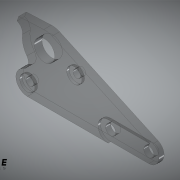
# Autodesk Inventor part: ロッド根本２
Saved by Autodesk Inventor 2020 (Build 240168000, 168)
## iProperties
Created: 2019-12-03
Part Number: ロッド根本２
Material: ポリカーボネート、クリア
Document SubType Name: Modeling
Designer: tanjihayato
Density: 1.2 g/cm^3
Appearance: ポリカーボネート - クリア
Mass: 2.90279 g
Surface Area: 23.7672 cm^2
Volume: 2.41899 cm^3
Author: tanjihayato
Autodesk Inventor part; units mm, degrees
ref_plane "YZ Plane" through (0, 0, 0) normal (1, 0, 0) x (0, 1, 0)
ref_plane "XZ Plane" through (0, 0, 0) normal (0, 1, 0) x (-1, 0, 0)
ref_plane "XY Plane" through (0, 0, 0) normal (0, 0, 1) x (1, 0, 0)
sketch "スケッチ2" plane through (0, 0, 0) normal (0, 0, 1) x (1, 0, 0)
  circle A0 centre (0, 0) radius 2
  circle A1 centre (15, 0) radius 2
  arc A2 (-0.2273, 4.9948) -> (-2.9263, -4.0542) centre (0, 0) ccw
  circle A3 centre (55, 0) radius 1.5
  circle A4 centre (55, 0) radius 4.025
  arc A5 (57.9262, 6.3865) -> (54.6807, 7.0177) centre (55, 0) ccw
  arc A6 (46.6204, -10.301) -> (48.0377, -5.2999) centre (45.4517, -7.2684) ccw
  circle A7 centre (95, -15) radius 2
  circle A8 centre (80, -15) radius 2
  arc A9 (95, -19) -> (96.6662, -11.3635) centre (95, -15) ccw
  line L0 (48.2385, -19) -> (80, -19)
  line L1 (57.9262, 6.3865) -> (96.6662, -11.3635)
  arc A10 (46.3293, 1.1755) -> (48.0377, -5.2999) centre (55, 0) ccw
  arc A11 (62.367, -1.4063) -> (54.6591, 7.4922) centre (55, 0) ccw
  line L2 (-0.2273, 4.9948) -> (54.6591, 7.4922)
  circle A12 centre (13, -10) radius 1.5
  arc A13 (10.3663, -13.6488) -> (12.3637, -14.4548) centre (13, -10) ccw
  line L3 (-2.9263, -4.0542) -> (10.3663, -13.6488)
  arc A14 (54.3637, -20.4538) -> (59.4202, -16.8428) centre (55, -15.999) ccw
  line L4 (12.3637, -14.4548) -> (54.3637, -20.4538)
  line L5 (59.4202, -16.8428) -> (62.367, -1.4063)
  circle A15 centre (66.7169, -2.5911) radius 1.5
  circle A16 centre (66.7169, -2.5911) radius 4.5 construction
  circle A17 centre (48.2385, -14.5) radius 1.5
  arc A18 (46.6204, -10.301) -> (48.2385, -19) centre (48.2385, -14.5) ccw
  line L6 (358.0202, -11) -> (380, -19)
  circle A19 centre (348.0202, -15) radius 1.25
  circle A20 centre (333.0202, -15) radius 1.25
  circle A21 centre (318.0202, -15) radius 1.25
  circle A22 centre (303.0202, -15) radius 1.25
  line L7 (80, -11) -> (207.8755, -11)
  line L8 (358.0202, -11) -> (248.9511, -11)
  arc A23 (213.7823, -10) -> (213.8378, -11) centre (210.8567, -10.6639) ccw
  line L9 (213.7823, -10) -> (214.7761, -9.8894)
  line L10 (213.8378, -11) -> (214.8378, -11)
  line L11 (219.357, -11) -> (218.357, -11)
  line L12 (218.2737, -9.5) -> (219.2676, -9.3894)
  line L13 (222.8762, -11) -> (223.8762, -11)
  line L14 (222.7652, -9) -> (223.7591, -8.8894)
  arc A24 (214.8378, -11) -> (218.357, -11) centre (216.5974, -10.3453) ccw
  arc A25 (218.2737, -9.5) -> (214.7761, -9.8894) centre (216.5974, -10.3453) ccw
  arc A26 (219.357, -11) -> (222.8762, -11) centre (221.1166, -10.0946) ccw
  arc A27 (222.7652, -9) -> (219.2676, -9.3894) centre (221.1166, -10.0946) ccw
  line L15 (210.8567, -10.6639) -> (233.0155, -9.4343) construction
  arc A28 (223.8762, -11) -> (229.892, -10.6107) centre (226.7628, -8.9308) ccw
  arc A29 (226.8407, -8.7739) -> (223.7591, -8.8894) centre (225.3075, -9.0352) ccw
  arc A30 (226.8407, -8.7739) -> (230.4998, -7.0068) centre (226.5478, -3.4953) ccw
  arc A31 (233.6316, -8.397) -> (230.4998, -7.0068) centre (231.2455, -9.5496) ccw
  arc A32 (235.4619, -12.6053) -> (229.892, -10.6107) centre (230.3136, -18.2076) ccw
  arc A33 (235.4619, -12.6053) -> (239.6511, -11) centre (234.0497, -2.6513) ccw
  arc A34 (259.6965, 4.4867) -> (265.8152, 14.9495) centre (248.2498, 18.2013) ccw
  arc A35 (220.191, -4.195) -> (265.8152, 14.9495) centre (219.3797, 61.6752) ccw
  line L16 (220.191, -4.195) -> (207.615, -4.3499)
  arc A36 (196.7777, -11) -> (207.615, -4.3499) centre (196.7777, 1.1554) ccw
  line L17 (222.8762, -11) -> (240.076, -10.0456) construction
  line L18 (222.7652, -9) -> (239.478, -8.0726) construction
  line L19 (239.6511, -11) -> (240.6511, -11)
  arc A37 (240.6511, -11) -> (242.7511, -11) centre (241.7011, -11) ccw
  line L20 (242.7511, -11) -> (243.7511, -11)
  arc A38 (243.7511, -11) -> (245.8511, -11) centre (244.8011, -11) ccw
  line L21 (245.8511, -11) -> (246.8511, -11)
  arc A39 (246.8511, -11) -> (248.9511, -11) centre (247.9011, -11) ccw
  arc A40 (240.735, -6.337) -> (238.7449, -7.0075) centre (239.7428, -6.6807) ccw
  arc A41 (243.5362, -5.2633) -> (241.5809, -6.0291) centre (242.5618, -5.6544) ccw
  arc A42 (246.2823, -4.0554) -> (244.3663, -4.9148) centre (245.3279, -4.4932) ccw
  arc A43 (248.9668, -2.7162) -> (247.0946, -3.6672) centre (248.0347, -3.1996) ccw
  arc A44 (233.6316, -8.397) -> (238.7449, -7.0075) centre (219.9279, 52.1342) ccw
  arc A45 (240.735, -6.337) -> (241.5809, -6.0291) centre (219.9279, 52.1342) ccw
  arc A46 (243.5362, -5.2633) -> (244.3663, -4.9148) centre (219.9279, 52.1342) ccw
  arc A47 (246.2823, -4.0554) -> (247.0946, -3.6672) centre (219.9279, 52.1342) ccw
  arc A48 (248.9668, -2.7162) -> (259.6965, 4.4867) centre (219.9279, 52.1342) ccw
  line L22 (196.7777, -11) -> (196.7777, -15)
  circle A49 centre (200.7777, -15) radius 1.25
  circle A50 centre (215.7777, -15) radius 1.25
  arc A51 (196.7777, -15) -> (200.7777, -19) centre (200.7777, -15) ccw
  arc A52 (215.7777, -19) -> (217.9536, -11.6436) centre (215.7777, -15) ccw
  circle A53 centre (200.7777, -15) radius 1.5
  circle A54 centre (215.7777, -15) radius 1.5
  line L23 (200.7777, -19) -> (215.7777, -19)
  circle A55 centre (45.4517, -7.2684) radius 1.5
  arc A56 (46.3293, 1.1755) -> (44.1782, 4.6812) centre (43.1088, 1.6121) ccw
  line L24 (54.6807, 7.0177) -> (44.8362, 6.5698)
  line L25 (44.8362, 6.5698) -> (44.1782, 4.6812)
  line L26 (80, -19) -> (95, -19)
  dimension "d81" = 4
  dimension "d82" = 4
  dimension "d83" = 15
  dimension "d84" = 3
  dimension "d85" = 3
  dimension "d86" = 8.05
  dimension "d87" = 3
  dimension "d88" = 6.5
  dimension "d89" = 4
  dimension "d90" = 4
  dimension "d91" = 15
  dimension "d92" = 15
  dimension "d93" = 3
  dimension "d94" = 3
  dimension "d95" = 3
  dimension "d96" = 40
  dimension "d97" = 40
  dimension "d98" = 15
  dimension "d99" = 13
  dimension "d100" = 3
  dimension "d101" = 3
  dimension "d102" = 3
  dimension "d104" = 380
  dimension "d106" = 4
  dimension "d108" = 2.5
  dimension "d109" = 2.5
  dimension "d110" = 2.5
  dimension "d111" = 2.5
  dimension "d113" = 15
  dimension "d114" = 15
  dimension "d115" = 15
  dimension "d116" = 10
  dimension "d117" = 6
  dimension "d118" = 1
  dimension "d119" = 1.5
  dimension "d120" = 1
  dimension "d121" = 1
  dimension "d122" = 1
  dimension "d123" = 2
  dimension "d124" = 1
  dimension "d125" = 1.0015
  dimension "d126" = 1.0015
  dimension "d127" = 0.7511
  dimension "d128" = 0.7511
  dimension "d129" = 3.176
  dimension "d130" = 3.176
  dimension "d131" = 1.05
  dimension "d132" = 1.05
  dimension "d133" = 1.05
  dimension "d134" = 1
  dimension "d135" = 1
  dimension "d136" = 1
  dimension "d137" = 2.1
  dimension "d138" = 2.1
  dimension "d139" = 2.1
  dimension "d140" = 2.1
  dimension "d141" = 3
  dimension "d142" = 3
  dimension "d143" = 3
  dimension "d144" = 2.5
  dimension "d145" = 2.5
  dimension "d146" = 15
  dimension "d148" = 8
  dimension "d149" = 8
  constraints: 87 point on circle, 57 centre point, 54 end point, 25 tangent, 13 point on line, 10 coincident, 8 horizontal, 7 collinear, 6 horizontal alignment, 2 concentric, 2 parallel, 1 vertical, 1 vertical alignment, 2 other
  measures "d81" diameter of A0
  measures "d82" diameter of A1
  measures "d83" distance of point (0, 0) A1.centre
  measures "d84" radial gap between concentric circles of A0 A2
  measures "d85" diameter of A3
  measures "d86" diameter of A4
  measures "d87" radial gap between concentric circles of A4 A5
  measures "d88" diameter of A6
  measures "d89" diameter of A7
  measures "d90" diameter of A8
  measures "d91" distance of A8.centre A7.centre
  measures "d92" diameter of A11
  measures "d93" diameter of A12
  measures "d94" radial gap between concentric circles of A12 A13
  measures "d95" diameter of A15
  measures "d96" distance of A4.centre A1.centre
  measures "d97" horizontal distance of A3.centre A7.centre
  measures "d98" vertical distance of A8.centre A3.centre
  measures "d99" horizontal distance of A12.centre point (0, 0)
  measures "d100" diameter of A17
  measures "d101" radial gap between concentric circles of A16 A15
  measures "d102" radial gap between concentric circles of A17 A18
  measures "d104" horizontal distance of point (0, 0) L6.end
  measures "d106" radius of A9
  measures "d108" diameter of A19
  measures "d109" diameter of A20
  measures "d110" diameter of A21
  measures "d111" diameter of A22
  measures "d113" distance of A21.centre A22.centre
  measures "d114" distance of A21.centre A20.centre
  measures "d115" distance of A19.centre A20.centre
  measures "d116" horizontal distance of A19.centre L6.start
  measures "d117" diameter of A23
  measures "d118" vertical distance of L10.start L9.start
  measures "d119" vertical distance of L11.end L12.start
  measures "d120" distance of L10.start L10.end
  measures "d121" distance of L11.end L11.start
  measures "d122" distance of L13.start L13.end
  measures "d123" vertical distance of L13.start L14.start
  measures "d124" distance of L14.start L14.end
  measures "d125" distance from line of L15 L14.start
  measures "d126" distance from line of L13.start L15
  measures "d127" distance from line of L15 L12.start
  measures "d128" distance from line of L15 L11.end
  measures "d129" angle of L14 L18
  measures "d130" angle of L13 L17
  measures "d131" radius of A37
  measures "d132" radius of A38
  measures "d133" radius of A39
  measures "d134" distance of L21.start L21.end
  measures "d135" distance of L20.start L20.end
  measures "d136" distance of L19.start L19.end
  measures "d137" diameter of A40
  measures "d138" diameter of A41
  measures "d139" diameter of A42
  measures "d140" diameter of A43
  measures "d141" distance of A40.centre A41.centre
  measures "d142" distance of A42.centre A41.centre
  measures "d143" distance of A43.centre A42.centre
  measures "d144" diameter of A49
  measures "d145" diameter of A50
  measures "d146" distance of A50.centre A49.centre
  measures "d148" diameter of A51
  measures "d149" diameter of A52
extrude "押し出し2" add sketch "スケッチ2" along normal blind 3 contours A11 L5 A14 L0 A18 A6 A10 A56 L25 L24 A5 L1 | L1 A9 L26 L0 A14 L5 A11
sketch "スケッチ3" plane through (0, 0, 3) normal (0, 0, 1) x (1, 0, 0)
  circle A0 centre (55, 0) radius 4.025 projected
  circle A1 centre (80, -15) radius 2 projected
  circle A2 centre (95, -15) radius 2 projected
  circle A3 centre (48.2385, -14.5) radius 1.5 projected
  circle A4 centre (66.7169, -2.5911) radius 1.5 projected
  arc A5 (57.9262, 6.3865) -> (54.6807, 7.0177) centre (55, 0) ccw projected
  line L0 (54.6807, 7.0177) -> (44.8362, 6.5698) projected
  line L1 (44.8362, 6.5698) -> (44.1782, 4.6812) projected
  arc A6 (46.3293, 1.1755) -> (44.1782, 4.6812) centre (43.1088, 1.6121) ccw projected
  arc A7 (46.3293, 1.1755) -> (48.0377, -5.2999) centre (55, 0) ccw projected
  arc A8 (46.6204, -10.301) -> (48.0377, -5.2999) centre (45.4517, -7.2684) ccw projected
  arc A9 (46.6204, -10.301) -> (48.2385, -19) centre (48.2385, -14.5) ccw projected
  line L2 (48.2385, -19) -> (95, -19) projected
  arc A10 (95, -19) -> (96.6662, -11.3635) centre (95, -15) ccw projected
  line L3 (96.6662, -11.3635) -> (57.9262, 6.3865) projected
  arc A11 (80, -11) -> (80, -19) centre (80, -15) ccw
  line L4 (80, -19) -> (95, -19)
  line L5 (48.2385, -19) -> (95, -19) projected
  line L6 (80, -11) -> (95.8727, -11)
  circle A12 centre (66.7169, -2.5911) radius 3
  circle A13 centre (48.2385, -14.5) radius 3
  point P0 (0, 0)
  dimension "d164" = 6
  dimension "d165" = 6
  constraints: 4 end point, 3 centre point, 3 coincident, 3 point on circle, 3 tangent, 2 horizontal, 2 point on line
  measures "d164" diameter of A12
  measures "d165" diameter of A13
extrude "押し出し3" cut sketch "スケッチ3" against normal blind 1 contours L3 A10 L2 A11 L6 | A12 | A13
sketch "スケッチ4" plane through (0, 0, 3) normal (0, 0, 1) x (1, 0, 0)
  circle A0 centre (95, -15) radius 2 projected
  circle A1 centre (80, -15) radius 2 projected
  arc A2 (95, -19) -> (96.6662, -11.3635) centre (95, -15) ccw projected
  line L0 (95.8727, -11) -> (96.6662, -11.3635) projected
  line L1 (80, -11) -> (95.8727, -11) projected
  arc A3 (80, -11) -> (80, -19) centre (80, -15) ccw projected
  line L2 (95, -19) -> (80, -19) projected
  circle A4 centre (55, 0) radius 4.025 projected
  circle A5 centre (80, -15) radius 2 projected
  circle A6 centre (95, -15) radius 2 projected
  circle A7 centre (48.2385, -14.5) radius 1.5 projected
  circle A8 centre (66.7169, -2.5911) radius 1.5 projected
  arc A9 (57.9262, 6.3865) -> (54.6807, 7.0177) centre (55, 0) ccw projected
  line L3 (96.6662, -11.3635) -> (57.9262, 6.3865) projected
  arc A10 (95, -19) -> (96.6662, -11.3635) centre (95, -15) ccw projected
  line L4 (48.2385, -19) -> (95, -19) projected
  arc A11 (46.6204, -10.301) -> (48.2385, -19) centre (48.2385, -14.5) ccw projected
  arc A12 (46.6204, -10.301) -> (48.0377, -5.2999) centre (45.4517, -7.2684) ccw projected
  arc A13 (46.3293, 1.1755) -> (48.0377, -5.2999) centre (55, 0) ccw projected
  arc A14 (46.3293, 1.1755) -> (44.1782, 4.6812) centre (43.1088, 1.6121) ccw projected
  line L5 (44.8362, 6.5698) -> (44.1782, 4.6812) projected
  line L6 (54.6807, 7.0177) -> (44.8362, 6.5698) projected
  circle A15 centre (66.7169, -2.5911) radius 3 projected
  circle A16 centre (48.2385, -14.5) radius 3 projected
  point P0 (0, 0)
equation "\"d126\" = d125"
equation "\"d128\" = d127"
equation "\"d130\" = d129"
